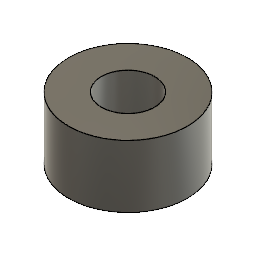
camera lens v1 (Autodesk Fusion 360 design; units mm, degrees)
Autodesk Fusion 360 part; units mm, degrees
sketch "Sketch1" plane through (0, 0, 0) normal (0, 1, 0) x (1, 0, 0)
  circle A0 centre (0, 0) radius 8.5
  circle A1 centre (0, 0) radius 9.5
  circle A2 centre (0, 0) radius 4.25
  dimension "d1" = 17
  dimension "d2" = 19
  dimension "d7" = 8.5
  measures "d1" diameter of A0
  measures "d2" diameter of A1
  measures "d7" diameter of A2
extrude "Extrude1" add sketch "Sketch1" along normal blind 20 contours A1
extrude "Extrude2" add sketch "Sketch1" along normal blind 20 contours A0 | A2
extrude "Extrude3" cut sketch "Sketch1" along normal blind 20 contours A2
extrude "Extrude4" cut 1 faces at (7.7146, 20, 0.472) along direction (0, -1, 0) blind 10
extrude "Extrude5" cut sketch "Sketch1" along normal blind 4 contours A0
